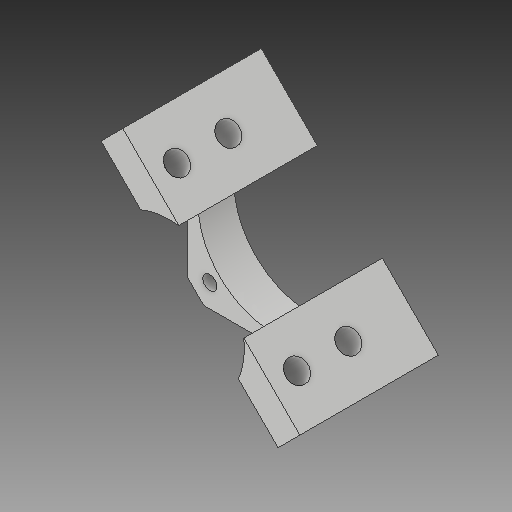
# Autodesk Inventor part: ZHolder
Saved by Autodesk Inventor 2019 (Build 230136000, 136)
## iProperties
Created: 2019-05-13
Part Number: ZHolder
Material: Generic
Document SubType Name: Modeling
Designer: Alex Jones
Density: 1 g/cm^3
Appearance: Default
Mass: 13.2763 g
Surface Area: 73.6151 cm^2
Volume: 13.2763 cm^3
Author: Alex Jones
Autodesk Inventor part; units mm, degrees
ref_plane "YZ Plane" through (0, 0, 0) normal (1, 0, 0) x (0, 1, 0)
ref_plane "XZ Plane" through (0, 0, 0) normal (0, 1, 0) x (-1, 0, 0)
ref_plane "XY Plane" through (0, 0, 0) normal (0, 0, 1) x (1, 0, 0)
sketch "Sketch1" plane through (0, 0, 0) normal (0, 0, 1) x (1, 0, 0)
  line L0 (-21.15, 16.8267) -> (-21.15, -16.8267) projected
  arc A0 (-21.15, -16.8267) -> (-21.0036, -17.1802) centre (-20.65, -16.8267) ccw projected
  line L1 (-21.0036, -17.1802) -> (-17.1802, -21.0036) projected
  arc A1 (-17.1802, -21.0036) -> (-16.8267, -21.15) centre (-16.8267, -20.65) ccw projected
  line L2 (-16.8267, -21.15) -> (16.8267, -21.15) projected
  arc A2 (16.8267, -21.15) -> (17.1802, -21.0036) centre (16.8267, -20.65) ccw projected
  line L3 (17.1802, -21.0036) -> (21.0036, -17.1802) projected
  arc A3 (21.0036, -17.1802) -> (21.15, -16.8267) centre (20.65, -16.8267) ccw projected
  line L4 (21.15, -16.8267) -> (21.15, 16.8267) projected
  arc A4 (21.15, 16.8267) -> (21.0036, 17.1802) centre (20.65, 16.8267) ccw projected
  line L5 (21.0036, 17.1802) -> (17.1802, 21.0036) projected
  arc A5 (17.1802, 21.0036) -> (16.8267, 21.15) centre (16.8267, 20.65) ccw projected
  line L6 (16.8267, 21.15) -> (-16.8267, 21.15) projected
  arc A6 (-16.8267, 21.15) -> (-17.1802, 21.0036) centre (-16.8267, 20.65) ccw projected
  line L7 (-17.1802, 21.0036) -> (-21.0036, 17.1802) projected
  arc A7 (-21.0036, 17.1802) -> (-21.15, 16.8267) centre (-20.65, 16.8267) ccw projected
  circle A8 centre (-15.5, -15.5) radius 1.75 projected
  circle A9 centre (-15.5, 15.5) radius 1.75 projected
  circle A10 centre (15.5, 15.5) radius 1.75 projected
  circle A11 centre (15.5, -15.5) radius 1.75 projected
  circle A12 centre (0, 0) radius 17 projected
  circle A13 centre (0, 0) radius 18.4295
  constraints: 1 centre point
extrude "Extrusion1" add sketch "Sketch1" along normal blind 8.89 contours A7 L7 A6 L6 A5 L5 A4 L4 A3 L3 A2 L2 A1 L1 A0 L0
sketch "Sketch2" plane through (0, 0, 8.89) normal (0, 0, 1) x (1, 0, 0)
  circle A0 centre (0, 0) radius 18.4295 projected
  circle A1 centre (15.5, -15.5) radius 1.75 projected
  circle A2 centre (15.5, 15.5) radius 1.75 projected
  circle A3 centre (-15.5, 15.5) radius 1.75 projected
  circle A4 centre (-15.5, -15.5) radius 1.75 projected
  line L0 (-21.15, 16.8267) -> (-21.15, -16.8267) projected
  arc A5 (-21.15, -16.8267) -> (-21.0036, -17.1802) centre (-20.65, -16.8267) ccw projected
  line L1 (-21.0036, -17.1802) -> (-17.1802, -21.0036) projected
  arc A6 (-17.1802, -21.0036) -> (-16.8267, -21.15) centre (-16.8267, -20.65) ccw projected
  line L2 (-16.8267, -21.15) -> (16.8267, -21.15) projected
  arc A7 (16.8267, -21.15) -> (17.1802, -21.0036) centre (16.8267, -20.65) ccw projected
  line L3 (17.1802, -21.0036) -> (21.0036, -17.1802) projected
  arc A8 (21.0036, -17.1802) -> (21.15, -16.8267) centre (20.65, -16.8267) ccw projected
  line L4 (21.15, -16.8267) -> (21.15, 16.8267) projected
  arc A9 (21.15, 16.8267) -> (21.0036, 17.1802) centre (20.65, 16.8267) ccw projected
  line L5 (21.0036, 17.1802) -> (17.1802, 21.0036) projected
  arc A10 (17.1802, 21.0036) -> (16.8267, 21.15) centre (16.8267, 20.65) ccw projected
  line L6 (16.8267, 21.15) -> (-16.8267, 21.15) projected
  arc A11 (-16.8267, 21.15) -> (-17.1802, 21.0036) centre (-16.8267, 20.65) ccw projected
  line L7 (-17.1802, 21.0036) -> (-21.0036, 17.1802) projected
  arc A12 (-21.0036, 17.1802) -> (-21.15, 16.8267) centre (-20.65, 16.8267) ccw projected
  arc A13 (15.7331, 31.2895) -> (15.7331, 33.0572) centre (14.8492, 32.1734) ccw projected
  line L8 (15.7331, 33.0572) -> (12.0915, 36.6988) projected
  line L9 (12.0915, 36.6988) -> (11.3844, 36.6988) projected
  line L10 (11.3844, 36.6988) -> (10.6066, 35.921) projected
  line L11 (10.6066, 35.921) -> (12.3037, 34.224) projected
  line L12 (12.3037, 34.224) -> (10.9361, 32.8564) projected
  line L13 (10.9361, 32.8564) -> (7.5901, 32.8564) projected
  line L14 (7.5901, 32.8564) -> (3.1579, 37.2886) projected
  line L15 (3.1579, 37.2886) -> (3.1579, 40.6346) projected
  line L16 (3.1579, 40.6346) -> (4.5255, 42.0021) projected
  line L17 (4.5255, 42.0021) -> (6.2225, 40.3051) projected
  line L18 (6.2225, 40.3051) -> (7.0004, 41.0829) projected
  line L19 (7.0004, 41.0829) -> (7.0004, 41.79) projected
  line L20 (7.0004, 41.79) -> (3.3588, 45.4316) projected
  arc A14 (3.3588, 45.4316) -> (1.591, 45.4316) centre (2.4749, 44.5477) ccw projected
  line L21 (1.591, 45.4316) -> (-2.0506, 41.79) projected
  line L22 (-2.0506, 41.79) -> (-2.0506, 41.0829) projected
  line L23 (-2.0506, 41.0829) -> (-1.2728, 40.3051) projected
  line L24 (-1.2728, 40.3051) -> (0.4243, 42.0021) projected
  line L25 (0.4243, 42.0021) -> (1.7918, 40.6346) projected
  line L26 (1.7918, 40.6346) -> (1.7918, 37.2886) projected
  line L27 (1.7918, 37.2886) -> (-2.6403, 32.8564) projected
  line L28 (-2.6403, 32.8564) -> (-5.9864, 32.8564) projected
  line L29 (-5.9864, 32.8564) -> (-7.3539, 34.224) projected
  line L30 (-7.3539, 34.224) -> (-5.6569, 35.921) projected
  line L31 (-5.6569, 35.921) -> (-6.4347, 36.6988) projected
  line L32 (-6.4347, 36.6988) -> (-7.1418, 36.6988) projected
  line L33 (-7.1418, 36.6988) -> (-10.7834, 33.0572) projected
  arc A15 (-10.7834, 33.0572) -> (-10.7834, 31.2895) centre (-9.8995, 32.1734) ccw projected
  line L34 (-10.7834, 31.2895) -> (-7.1418, 27.6479) projected
  line L35 (-7.1418, 27.6479) -> (-6.4347, 27.6479) projected
  line L36 (-6.4347, 27.6479) -> (-5.6569, 28.4257) projected
  line L37 (-5.6569, 28.4257) -> (-7.3539, 30.1228) projected
  line L38 (-7.3539, 30.1228) -> (-5.9864, 31.4903) projected
  line L39 (-5.9864, 31.4903) -> (-2.6403, 31.4903) projected
  line L40 (-2.6403, 31.4903) -> (1.7918, 27.0582) projected
  line L41 (1.7918, 27.0582) -> (1.7918, 23.7121) projected
  line L42 (1.7918, 23.7121) -> (0.4243, 22.3446) projected
  line L43 (0.4243, 22.3446) -> (-1.2728, 24.0416) projected
  line L44 (-1.2728, 24.0416) -> (-2.0506, 23.2638) projected
  line L45 (-2.0506, 23.2638) -> (-2.0506, 22.5567) projected
  line L46 (-2.0506, 22.5567) -> (1.591, 18.9151) projected
  arc A16 (1.591, 18.9151) -> (3.3588, 18.9151) centre (2.4749, 19.799) ccw projected
  line L47 (3.3588, 18.9151) -> (7.0004, 22.5567) projected
  line L48 (7.0004, 22.5567) -> (7.0004, 23.2638) projected
  line L49 (7.0004, 23.2638) -> (6.2225, 24.0416) projected
  line L50 (6.2225, 24.0416) -> (4.5255, 22.3446) projected
  line L51 (4.5255, 22.3446) -> (3.1579, 23.7121) projected
  line L52 (3.1579, 23.7121) -> (3.1579, 27.0582) projected
  line L53 (3.1579, 27.0582) -> (7.5901, 31.4903) projected
  line L54 (7.5901, 31.4903) -> (10.9361, 31.4903) projected
  line L55 (10.9361, 31.4903) -> (12.3037, 30.1228) projected
  line L56 (12.3037, 30.1228) -> (10.6066, 28.4257) projected
  line L57 (10.6066, 28.4257) -> (11.3844, 27.6479) projected
  line L58 (11.3844, 27.6479) -> (12.0915, 27.6479) projected
  line L59 (12.0915, 27.6479) -> (15.7331, 31.2895) projected
  circle A17 centre (2.4749, 32.1734) radius 2.5 projected
  arc A18 (45.4316, 1.591) -> (45.4316, 3.3588) centre (44.5477, 2.4749) ccw projected
  line L60 (45.4316, 3.3588) -> (41.79, 7.0004) projected
  line L61 (41.79, 7.0004) -> (41.0829, 7.0004) projected
  line L62 (41.0829, 7.0004) -> (40.3051, 6.2225) projected
  line L63 (40.3051, 6.2225) -> (42.0021, 4.5255) projected
  line L64 (42.0021, 4.5255) -> (40.6346, 3.158) projected
  line L65 (40.6346, 3.158) -> (37.2886, 3.158) projected
  line L66 (37.2886, 3.158) -> (32.8564, 7.5901) projected
  line L67 (32.8564, 7.5901) -> (32.8564, 10.9361) projected
  line L68 (32.8564, 10.9361) -> (34.224, 12.3037) projected
  line L69 (34.224, 12.3037) -> (35.921, 10.6066) projected
  line L70 (35.921, 10.6066) -> (36.6988, 11.3844) projected
  line L71 (36.6988, 11.3844) -> (36.6988, 12.0915) projected
  line L72 (36.6988, 12.0915) -> (33.0572, 15.7331) projected
  arc A19 (33.0572, 15.7331) -> (31.2895, 15.7331) centre (32.1734, 14.8492) ccw projected
  line L73 (31.2895, 15.7331) -> (27.6479, 12.0915) projected
  line L74 (27.6479, 12.0915) -> (27.6479, 11.3844) projected
  line L75 (27.6479, 11.3844) -> (28.4257, 10.6066) projected
  line L76 (28.4257, 10.6066) -> (30.1227, 12.3037) projected
  line L77 (30.1227, 12.3037) -> (31.4903, 10.9361) projected
  line L78 (31.4903, 10.9361) -> (31.4903, 7.5901) projected
  line L79 (31.4903, 7.5901) -> (27.0582, 3.158) projected
  line L80 (27.0582, 3.158) -> (23.7121, 3.158) projected
  line L81 (23.7121, 3.158) -> (22.3446, 4.5255) projected
  line L82 (22.3446, 4.5255) -> (24.0416, 6.2225) projected
  line L83 (24.0416, 6.2225) -> (23.2638, 7.0004) projected
  line L84 (23.2638, 7.0004) -> (22.5567, 7.0004) projected
  line L85 (22.5567, 7.0004) -> (18.9151, 3.3588) projected
  arc A20 (18.9151, 3.3588) -> (18.9151, 1.591) centre (19.799, 2.4749) ccw projected
  line L86 (18.9151, 1.591) -> (22.5567, -2.0506) projected
  line L87 (22.5567, -2.0506) -> (23.2638, -2.0506) projected
  line L88 (23.2638, -2.0506) -> (24.0416, -1.2728) projected
  line L89 (24.0416, -1.2728) -> (22.3446, 0.4243) projected
  line L90 (22.3446, 0.4243) -> (23.7121, 1.7918) projected
  line L91 (23.7121, 1.7918) -> (27.0582, 1.7918) projected
  line L92 (27.0582, 1.7918) -> (31.4903, -2.6403) projected
  line L93 (31.4903, -2.6403) -> (31.4903, -5.9864) projected
  line L94 (31.4903, -5.9864) -> (30.1227, -7.3539) projected
  line L95 (30.1227, -7.3539) -> (28.4257, -5.6569) projected
  line L96 (28.4257, -5.6569) -> (27.6479, -6.4347) projected
  line L97 (27.6479, -6.4347) -> (27.6479, -7.1418) projected
  line L98 (27.6479, -7.1418) -> (31.2895, -10.7834) projected
  arc A21 (31.2895, -10.7834) -> (33.0572, -10.7834) centre (32.1734, -9.8995) ccw projected
  line L99 (33.0572, -10.7834) -> (36.6988, -7.1418) projected
  line L100 (36.6988, -7.1418) -> (36.6988, -6.4347) projected
  line L101 (36.6988, -6.4347) -> (35.921, -5.6569) projected
  line L102 (35.921, -5.6569) -> (34.224, -7.3539) projected
  line L103 (34.224, -7.3539) -> (32.8564, -5.9864) projected
  line L104 (32.8564, -5.9864) -> (32.8564, -2.6403) projected
  line L105 (32.8564, -2.6403) -> (37.2886, 1.7918) projected
  line L106 (37.2886, 1.7918) -> (40.6346, 1.7918) projected
  line L107 (40.6346, 1.7918) -> (42.0021, 0.4243) projected
  line L108 (42.0021, 0.4243) -> (40.3051, -1.2728) projected
  line L109 (40.3051, -1.2728) -> (41.0829, -2.0506) projected
  line L110 (41.0829, -2.0506) -> (41.79, -2.0506) projected
  line L111 (41.79, -2.0506) -> (45.4316, 1.591) projected
  circle A22 centre (32.1734, 2.4749) radius 2.5 projected
  line L112 (0, 0) -> (0, 42.5275)
  line L113 (17.1802, -21.0036) -> (21.0036, -17.1802) projected
  line L114 (17.1802, -21.0036) -> (32.1734, -11.6673)
  line L115 (32.1734, -11.6673) -> (21.15, -0.6439)
  line L116 (21.15, -16.8267) -> (21.15, 16.8267) projected
  line L117 (21.15, -0.6439) -> (17.1802, -21.0036)
  line L118 (0, 0) -> (48.328, 48.328)
  line L119 (-21.0036, 17.1802) -> (-11.6673, 32.1734)
  line L120 (-11.6673, 32.1734) -> (-0.6439, 21.15)
  line L121 (-0.6439, 21.15) -> (-21.0036, 17.1802)
  constraints: 16 end point, 3 point on line, 2 symmetric about line, 1 vertical
extrude "Extrusion2" add sketch "Sketch2" against normal up to surface (8.89 mm away) contours L121 L7 A11 L6 | L6 A11 L7 L119 L120 L34 L46 | L86 L115 L98 L114 L3 A8 L4 | L4 A8 L3 L117
sketch "Sketch3" plane through (0, 0, 8.89) normal (0, 0, 1) x (1, 0, 0)
  arc A0 (-21.0036, 17.1802) -> (-21.15, 16.8267) centre (-20.65, 16.8267) ccw projected
  line L0 (-21.15, 16.8267) -> (-21.15, -16.8267) projected
  arc A1 (-21.15, -16.8267) -> (-21.0036, -17.1802) centre (-20.65, -16.8267) ccw projected
  line L1 (-21.0036, -17.1802) -> (-17.1802, -21.0036) projected
  arc A2 (-17.1802, -21.0036) -> (-16.8267, -21.15) centre (-16.8267, -20.65) ccw projected
  line L2 (-16.8267, -21.15) -> (16.8267, -21.15) projected
  arc A3 (16.8267, -21.15) -> (17.1802, -21.0036) centre (16.8267, -20.65) ccw projected
  line L3 (17.1802, -21.0036) -> (32.1734, -11.6673) projected
  line L4 (32.1734, -11.6673) -> (21.15, -0.6439) projected
  line L5 (21.15, -0.6439) -> (21.15, 16.8267) projected
  arc A4 (21.15, 16.8267) -> (21.0036, 17.1802) centre (20.65, 16.8267) ccw projected
  line L6 (21.0036, 17.1802) -> (17.1802, 21.0036) projected
  arc A5 (17.1802, 21.0036) -> (16.8267, 21.15) centre (16.8267, 20.65) ccw projected
  line L7 (16.8267, 21.15) -> (-0.6439, 21.15) projected
  line L8 (-0.6439, 21.15) -> (-11.6673, 32.1734) projected
  line L9 (-11.6673, 32.1734) -> (-21.0036, 17.1802) projected
  circle A6 centre (0, 0) radius 18.4295 projected
  circle A7 centre (15.5, -15.5) radius 1.75 projected
  circle A8 centre (15.5, 15.5) radius 1.75 projected
  circle A9 centre (-15.5, 15.5) radius 1.75 projected
  circle A10 centre (-15.5, -15.5) radius 1.75 projected
  line L10 (21.15, -0.6439) -> (32.1734, -11.6673) projected
  line L11 (32.1734, -11.6673) -> (18.0312, 2.4749)
  line L12 (18.0312, 2.4749) -> (12.6431, -2.9133)
  line L13 (12.6431, -2.9133) -> (26.7852, -17.0554)
  line L14 (26.7852, -17.0554) -> (32.1734, -11.6673)
  line L15 (0, 0) -> (-64.6298, -64.6298)
  line L16 (-11.6673, 32.1734) -> (-0.6439, 21.15)
  line L17 (-0.6439, 21.15) -> (-11.6673, 32.1734)
  line L18 (-11.6673, 32.1734) -> (2.4749, 18.0312)
  line L19 (2.4749, 18.0312) -> (-2.9133, 12.6431)
  line L20 (-2.9133, 12.6431) -> (-17.0554, 26.7852)
  line L21 (-17.0554, 26.7852) -> (-11.6673, 32.1734)
  dimension "d5" = 7.62
  dimension "d6" = 20
  constraints: 22 end point, 3 symmetric about line, 2 parallel, 2 point on line, 1 perpendicular
  measures "d5" distance of L13.end L3.end
  measures "d6" distance of L12.end L13.end
extrude "Extrusion3" add sketch "Sketch3" along normal blind 25.4 contours L20 L21 L9 | L9 L8 L18 A6 L20 | A6 L18 L19 L20 | L11 L4 L3 L13 A6 | A6 L13 L12 L11 | L3 L14 L13
sketch "Sketch4" plane through (0, 0, 8.89) normal (0, 0, 1) x (1, 0, 0)
  line L0 (-7.2246, 16.9544) -> (-15.8026, 25.5324) projected
  line L1 (-15.8026, 25.5324) -> (-21.0036, 17.1802) projected
  arc A0 (-21.0036, 17.1802) -> (-21.15, 16.8267) centre (-20.65, 16.8267) ccw projected
  line L2 (-21.15, 16.8267) -> (-21.15, -16.8267) projected
  arc A1 (-21.15, -16.8267) -> (-21.0036, -17.1802) centre (-20.65, -16.8267) ccw projected
  line L3 (-21.0036, -17.1802) -> (-17.1802, -21.0036) projected
  arc A2 (-17.1802, -21.0036) -> (-16.8267, -21.15) centre (-16.8267, -20.65) ccw projected
  line L4 (-16.8267, -21.15) -> (16.8267, -21.15) projected
  arc A3 (16.8267, -21.15) -> (17.1802, -21.0036) centre (16.8267, -20.65) ccw projected
  line L5 (17.1802, -21.0036) -> (25.5324, -15.8026) projected
  line L6 (25.5324, -15.8026) -> (16.9544, -7.2246) projected
  arc A4 (-7.2246, 16.9544) -> (16.9544, -7.2246) centre (0, 0) ccw projected
  circle A5 centre (15.5, -15.5) radius 1.75 projected
  circle A6 centre (-15.5, 15.5) radius 1.75 projected
  circle A7 centre (-15.5, -15.5) radius 1.75 projected
  line L7 (25.5324, -15.8026) -> (32.1734, -11.6673) projected
  line L8 (32.1734, -11.6673) -> (18.0312, 2.4749) projected
  line L9 (18.0312, 2.4749) -> (12.6431, -2.9133) projected
  line L10 (12.6431, -2.9133) -> (26.7852, -17.0554) projected
  line L11 (26.7852, -17.0554) -> (32.1734, -11.6673) projected
  line L12 (-11.6673, 32.1734) -> (-17.0554, 26.7852) projected
  line L13 (-17.0554, 26.7852) -> (-2.9133, 12.6431) projected
  line L14 (-2.9133, 12.6431) -> (2.4749, 18.0312) projected
  line L15 (2.4749, 18.0312) -> (-11.6673, 32.1734) projected
  line L16 (17.1802, -21.0036) -> (20.0086, -23.832)
  line L17 (21.15, -0.6439) -> (32.1734, -11.6673) projected
  line L18 (32.1734, -11.6673) -> (20.0086, -23.832)
  line L19 (32.1734, -11.6673) -> (17.1802, -21.0036) projected
  line L20 (17.1802, -21.0036) -> (32.1734, -11.6673)
  line L21 (0, 0) -> (-37.9127, -37.9127)
  arc A8 (-21.0036, 17.1802) -> (-21.15, 16.8267) centre (-20.65, 16.8267) ccw
  line L22 (-21.0036, 17.1802) -> (-15.8026, 25.5324)
  line L23 (-15.8026, 25.5324) -> (-11.6673, 32.1734)
  line L24 (-17.0554, 26.7852) -> (-11.6673, 32.1734)
  line L25 (-21.0036, 17.1802) -> (-23.832, 20.0086)
  line L26 (-11.6673, 32.1734) -> (-23.832, 20.0086)
  line L27 (-11.6673, 32.1734) -> (-21.0036, 17.1802)
  line L28 (-21.0036, 17.1802) -> (-11.6673, 32.1734)
  constraints: 22 end point, 4 symmetric about line, 2 point on circle, 1 centre point, 1 collinear, 1 perpendicular, 1 other
extrude "Extrusion4" add sketch "Sketch4" against normal up to surface (8.89 mm away) contours L1 L25 L26 L13 | L13 L12 L23 | L10 L18 L16 L5 | L7 L11 L10
sketch "Sketch5" plane through (0, 0, 8.89) normal (0, 0, 1) x (1, 0, 0)
  circle A0 centre (15.5, 15.5) radius 1.75 projected
  line L0 (-0.6439, 21.15) -> (2.2095, 18.2966) projected
  arc A1 (18.2966, 2.2095) -> (2.2095, 18.2966) centre (0, 0) ccw projected
  line L1 (18.2966, 2.2095) -> (21.15, -0.6439) projected
  line L2 (21.15, -0.6439) -> (21.15, 16.8267) projected
  arc A2 (21.15, 16.8267) -> (21.0036, 17.1802) centre (20.65, 16.8267) ccw projected
  line L3 (21.0036, 17.1802) -> (17.1802, 21.0036) projected
  arc A3 (17.1802, 21.0036) -> (16.8267, 21.15) centre (16.8267, 20.65) ccw projected
  line L4 (16.8267, 21.15) -> (-0.6439, 21.15) projected
extrude "Extrusion5" cut sketch "Sketch5" against normal blind 25.4
sketch "Sketch6" plane through (32.1734, -11.6673, 34.29) normal (0.7071068, -0.7071068, 0) x (-0.7071068, -0.7071068, 0)
  line L0 (0, 34.29) -> (0, 0) projected
  line L1 (7.62, 0) -> (0, 0) projected
  line L2 (7.62, 25.4) -> (7.62, 0) projected
  line L3 (17.2035, 25.4) -> (7.62, 25.4) projected
  line L4 (17.2035, 25.4) -> (17.2035, 34.29) projected
  line L5 (0, 34.29) -> (17.2035, 34.29) projected
  line L6 (7.62, 25.4) -> (7.62, 0) projected
  line L7 (7.62, 0) -> (17.2035, 25.4)
  line L8 (32.9295, 25.4) -> (7.62, 25.4) projected
  line L9 (17.2035, 25.4) -> (7.62, 25.4)
  line L10 (0, 0) -> (7.62, 0) projected
  line L11 (7.62, 25.4) -> (7.62, 0)
  point P0 (14.5, 34.29)
  constraints: 6 end point, 1 horizontal, 1 perpendicular
extrude "Extrusion6" add sketch "Sketch6" against normal blind 3.81 contours L2 L3 L7
sketch "Sketch7" plane through (-11.6673, 32.1734, 0) normal (-0.7071068, 0.7071068, 0) x (-0.7071068, -0.7071068, 0)
  line L0 (17.2035, 8.89) -> (7.62, 34.29) projected
  line L1 (7.62, 8.89) -> (7.62, 34.29) projected
  line L2 (17.2035, 8.89) -> (7.62, 8.89) projected
  point P0 (14.5, 0)
extrude "Extrusion7" add sketch "Sketch7" against normal blind 3.81
sketch "Sketch8" plane through (12.6431, -2.9133, 34.29) normal (-0.7071068, -0.7071068, 0) x (-0.7071068, 0.7071068, 0)
  line L0 (-20, 0) -> (-20, 25.4) projected
  line L1 (0, 25.4) -> (0, 0) projected
  line L2 (22, 25.4) -> (22, 0) projected
  line L3 (42, 25.4) -> (42, 0) projected
  line L4 (22, 12.7) -> (42, 12.7) construction
  line L5 (42, 34.29) -> (42, 0) projected
  line L6 (-20, 12.7) -> (0, 12.7) construction
  line L7 (-10, 12.7) -> (-10, 0) construction
  line L8 (-20, 0) -> (0, 0) projected
  line L9 (32, 12.7) -> (32, 0) construction
  line L10 (22, 0) -> (42, 0) projected
  line L11 (32, 12.7) -> (32, 25.4) construction
  line L12 (31.1703, 34.29) -> (31.1703, 25.4) projected
  line L13 (-10, 12.7) -> (-10, 25.4) construction
  circle A0 centre (-10, 19.05) radius 2.75
  circle A1 centre (-10, 6.35) radius 2.75
  circle A2 centre (32, 6.35) radius 2.75
  circle A3 centre (32, 19.05) radius 2.75
  point P0 (11, 34.29)
  dimension "d17" = 5.5
  constraints: 12 end point, 11 midpoint, 4 centre point, 3 equal radius, 1 horizontal, 1 parallel, 1 point on line, 1 vertical
  measures "d17" diameter of A0
extrude "Extrusion8" cut sketch "Sketch8" against normal through all
sketch "Sketch9" plane through (0, 0, 8.89) normal (0, 0, -1) x (-1, 0, 0)
  arc A0 (-18.2966, 2.2095) -> (-16.9544, -7.2246) centre (0, 0) ccw projected
  line L0 (-12.6431, -2.9133) -> (-16.9544, -7.2246) projected
  line L1 (-18.0312, 2.4749) -> (-12.6431, -2.9133) projected
  line L2 (-18.2966, 2.2095) -> (-18.0312, 2.4749) projected
  arc A1 (7.2246, 16.9544) -> (-2.2095, 18.2966) centre (0, 0) ccw projected
  line L3 (-2.4749, 18.0312) -> (-2.2095, 18.2966) projected
  line L4 (2.9133, 12.6431) -> (-2.4749, 18.0312) projected
  line L5 (7.2246, 16.9544) -> (2.9133, 12.6431) projected
extrude "Extrusion9" cut sketch "Sketch9" against normal through all
body "Solid1"
